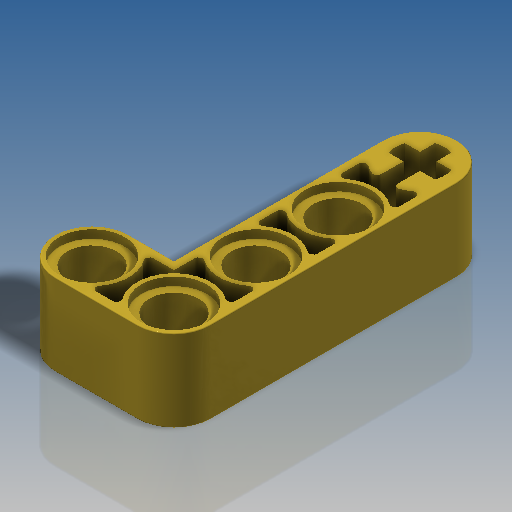
# Autodesk Inventor part: 32140-Yellow
Saved by Autodesk Inventor 2018.3 (Build 223284000, 284)
## iProperties
Created: 2012-03-21
Part Number: 32140-Yellow
Document SubType Name: Modeling
Designer: D. Kohfeld
Density: 1.06 g/cm^3
Material: ABS Plastic
Mass: 1.20524 g
Surface Area: 20.9457 cm^2
Volume: 1.13702 cm^3
Appearance: Yellow
Author: D. Kohfeld
Autodesk Inventor part; units mm, degrees
ref_plane "YZ Plane" through (0, 0, 0) normal (1, 0, 0) x (0, 1, 0)
ref_plane "XZ Plane" through (0, 0, 0) normal (0, 1, 0) x (-1, 0, 0)
ref_plane "XY Plane" through (0, 0, 0) normal (0, 0, 1) x (1, 0, 0)
sketch "Sketch1" plane through (0, 0, 0) normal (0, 0, 1) x (1, 0, 0)
  line L0 (3.6, -12) -> (3.6, 12)
  line L1 (-3.6, 12) -> (-3.6, -8.4)
  arc A0 (3.6, 12) -> (-3.6, 12) centre (0, 12) ccw
  circle A1 centre (0, 4) radius 2.4
  circle A2 centre (0, 4) radius 3.2
  circle A3 centre (0, -4) radius 3.2
  circle A4 centre (0, -4) radius 2.4
  line L2 (0, -4) -> (0, 4) construction
  line L3 (-2.8, 1.7373) -> (-2.8, -1.7373)
  line L4 (2.8, 1.7373) -> (2.8, -1.7373)
  arc A5 (-2.8, 1.7373) -> (2.8, 1.7373) centre (0, 4) ccw
  arc A6 (2.8, -1.7373) -> (-2.8, -1.7373) centre (0, -4) ccw
  circle A7 centre (0, -12) radius 3.2
  circle A8 centre (0, -12) radius 2.4
  line L5 (0, -4) -> (0, -12) construction
  line L6 (-2.8, -6.2627) -> (-2.8, -9.7373)
  line L7 (2.8, -6.2627) -> (2.8, -9.7373)
  arc A9 (-2.8, -6.2627) -> (2.8, -6.2627) centre (0, -4) ccw
  arc A10 (2.8, -9.7373) -> (-2.8, -9.7373) centre (0, -12) ccw
  circle A11 centre (0, 12) radius 2.4 construction
  line L8 (0, 12) -> (0, 4) construction
  line L9 (2.8, 9.7373) -> (2.8, 6.2627)
  line L10 (-2.8, 9.7373) -> (-2.8, 6.2627)
  arc A12 (-2.8, 9.7373) -> (2.8, 9.7373) centre (0, 12) ccw
  arc A13 (2.8, 6.2627) -> (-2.8, 6.2627) centre (0, 4) ccw
  line L11 (-3.6, -8.4) -> (-8, -8.4)
  arc A14 (-8, -8.4) -> (-8, -15.6) centre (-8, -12) ccw
  line L12 (-8, -15.6) -> (0, -15.6)
  arc A15 (0, -15.6) -> (3.6, -12) centre (0, -12) ccw
  circle A16 centre (-8, -12) radius 3.2
  circle A17 centre (-8, -12) radius 2.4
  line L13 (-8, -12) -> (0, -12) construction
  line L14 (-0.8, 14.2627) -> (-0.8, 12.8)
  line L15 (-0.8, 12.8) -> (-2.2627, 12.8)
  line L16 (-2.2627, 11.2) -> (-0.8, 11.2)
  line L17 (-0.8, 11.2) -> (-0.8, 8.49)
  line L18 (0.8, 8.49) -> (0.8, 11.2)
  line L19 (0.8, 11.2) -> (2.2627, 11.2)
  line L20 (2.2627, 12.8) -> (0.8, 12.8)
  line L21 (0.8, 12.8) -> (0.8, 14.2627)
  arc A18 (0.8, 14.2627) -> (-0.8, 14.2627) centre (0, 12) ccw
  arc A19 (-2.2627, 12.8) -> (-2.2627, 11.2) centre (0, 12) ccw
  arc A20 (2.2627, 11.2) -> (2.2627, 12.8) centre (0, 12) ccw
  line L22 (-5.7373, -9.2) -> (-2.2627, -9.2)
  line L23 (-5.7373, -14.8) -> (-2.2627, -14.8)
  arc A21 (-5.7373, -14.8) -> (-5.7373, -9.2) centre (-8, -12) ccw
  arc A22 (-2.2627, -9.2) -> (-2.2627, -14.8) centre (0, -12) ccw
  point P0 (0, 0)
  point P1 (0, 0)
  dimension "d8" = 4.8
  dimension "d9" = 6.4
  dimension "d32" = 7.2
  dimension "d34" = 8
  dimension "d36" = 0.8
  dimension "d48" = 1.6
  dimension "d49" = 0.8
  constraints: 48 end point, 36 point on circle, 23 centre point, 20 equal radius, 15 coincident, 14 equal length, 13 parallel, 7 perpendicular, 5 tangent, 3 vertical, 2 concentric, 2 vertical alignment, 1 midpoint
  measures "d8" diameter of A1
  measures "d9" diameter of A2
  measures "d32" diameter of A0
  measures "d34" distance of L2.start L2.end
  measures "d36" distance between parallel lines of L1 L3
  measures "d48" distance between parallel lines of L21 L14
  measures "d49" distance between parallel lines of L11 L22
extrude "Extrusion1" add sketch "Sketch1" along normal mid plane 8 contours A15 L12 A14 L11 L1 A0 L0 | A2 | A3 | A5 L4 A6 L3 | A7 | A9 L7 A10 L22 L6 | L22 A10 L6 | L6 A22 L23 A21 L22 | A16
sketch "Sketch6" plane through (0, 0, 4) normal (0, 0, 1) x (1, 0, 0)
  circle A0 centre (0, -4) radius 3.2 projected
  circle A1 centre (0, 4) radius 3.2 projected
  arc A2 (2.8, -1.7373) -> (-2.8, -1.7373) centre (0, -4) ccw projected
  line L0 (-2.8, 1.7373) -> (-2.8, -1.7373) projected
  arc A3 (-2.8, 1.7373) -> (2.8, 1.7373) centre (0, 4) ccw projected
  line L1 (2.8, 1.7373) -> (2.8, -1.7373) projected
  line L2 (-2.8, -6.2627) -> (-2.8, -9.7373) projected
  arc A4 (-2.8, -6.2627) -> (2.8, -6.2627) centre (0, -4) ccw projected
  arc A5 (2.8, -9.7373) -> (-2.8, -9.7373) centre (0, -12) ccw projected
  line L3 (2.8, -6.2627) -> (2.8, -9.7373) projected
  circle A6 centre (0, -12) radius 3.2 projected
  circle A7 centre (0, -12) radius 2.4 projected
  line L4 (2.8, 9.7373) -> (2.8, 6.2627) projected
  arc A8 (-2.8, 9.7373) -> (2.8, 9.7373) centre (0, 12) ccw projected
  arc A9 (2.8, 6.2627) -> (-2.8, 6.2627) centre (0, 4) ccw projected
  line L5 (-2.8, 9.7373) -> (-2.8, 6.2627) projected
  line L6 (-5.7373, -9.2) -> (-2.2627, -9.2) projected
  arc A10 (-5.7373, -14.8) -> (-5.7373, -9.2) centre (-8, -12) ccw projected
  arc A11 (-2.2627, -9.2) -> (-2.2627, -14.8) centre (0, -12) ccw projected
  line L7 (-5.7373, -14.8) -> (-2.2627, -14.8) projected
  circle A12 centre (-8, -12) radius 3.2 projected
extrude "Extrusion7" cut sketch "Sketch6" against normal blind 0.8 contours A0 | A1 | A6 | A7 | A12
extrude "Extrusion8" cut sketch "Sketch6" against normal blind 3.1 contours A2 L0 A3 L1 | A4 L3 A5 L6 L2 | L6 A5 L2 | L2 A11 L7 A10 L6 | L4 A9 L5 A8
mirror "Mirror1" about plane through (0, 0, 0) normal (0, 0, 1) of "Extrusion7", "Extrusion8"
fillet "Fillet1" radius 0.4 26 edges at (-2.8, -1.7373, 2.45) (-2.8, 1.7373, 2.45) (2.8, -1.7373, 2.45) (2.8, 1.7373, 2.45) (2.8, 1.7373, -2.45) (2.8, -1.7373, -2.45) (-2.8, -1.7373, -2.45) (-2.8, 1.7373, -2.45) (-2.8, -6.2627, 2.45) (2.8, -9.7373, 2.45) (2.8, -6.2627, 2.45) (2.8, -6.2627, -2.45) (2.8, -9.7373, -2.45) (-2.8, -6.2627, -2.45) (-2.8, 6.2627, 0) (-2.8, 9.7373, 0) (-0.8, 8.49, 0) (0.8, 8.49, 0) (2.8, 9.7373, 0) (2.8, 6.2627, 0) (-5.7373, -9.2, 2.45) (-5.7373, -14.8, 2.45) (-2.2627, -14.8, 2.45) (-5.7373, -14.8, -2.45) (-2.2627, -14.8, -2.45) (-5.7373, -9.2, -2.45)
fillet "Fillet1" radius 0.1 6 edges at (-3.6, 1.8, 4) (0, 15.6, 4) (3.6, 0, 4) (0, 15.6, -4) (-3.6, 1.8, -4) (3.6, 0, -4)
body "Solid1"
